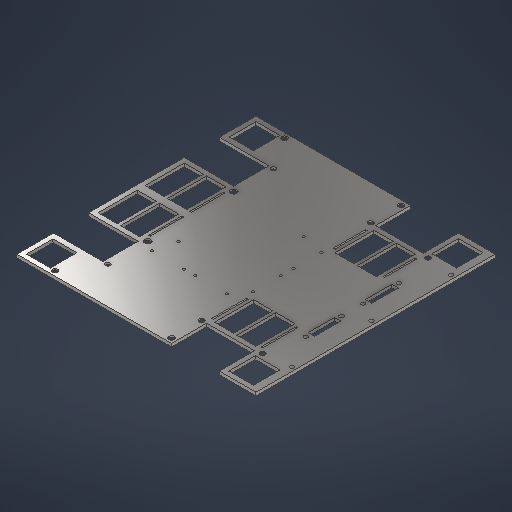
# Autodesk Inventor part: base
Saved by Autodesk Inventor 2026.2 (Build 302298010, 298A)
## iProperties
Created: 2026-04-27
Part Number: base
Material: Steel, Mild
Document SubType Name: Modeling
Designer: karol
Density: 7.85 g/cm^3
Appearance: Semi-Polished
Mass: 32.7977 g
Surface Area: 363.268 cm^2
Volume: 32.7977 cm^3
Author: karol
Autodesk Inventor part; units mm, degrees
ref_plane "YZ Plane" through (0, 0, 0) normal (1, 0, 0) x (0, 1, 0)
ref_plane "XZ Plane" through (0, 0, 0) normal (0, 1, 0) x (-1, 0, 0)
ref_plane "XY Plane" through (0, 0, 0) normal (0, 0, 1) x (1, 0, 0)
sketch "Szkic1" plane through (0, 0, 0) normal (0, 1, 0) x (-1, 0, 0)
  line L0 (0, 0) -> (150, 0)
  line L1 (150, 0) -> (150, -75)
  line L2 (150, -75) -> (0, -75)
  line L3 (0, -75) -> (0, 0)
  line L4 (53, -53) -> (23, -53)
  line L5 (23, -53) -> (23, -75)
  line L6 (23, -75) -> (53, -75)
  line L7 (53, -75) -> (53, -53)
  line L8 (23, -53) -> (20, -53)
  line L9 (20, -53) -> (20, -75)
  line L10 (20, -75) -> (23, -75)
  line L11 (23, -75) -> (23, -53)
  line L12 (20, -75) -> (0, -75)
  line L13 (0, -75) -> (0, -72)
  line L14 (0, -72) -> (20, -72)
  line L15 (20, -72) -> (20, -75)
  line L16 (20, -72) -> (5, -72)
  line L17 (5, -72) -> (5, -55.8)
  line L18 (5, -55.8) -> (20, -55.8)
  line L19 (20, -55.8) -> (20, -72)
  line L20 (150, 0) -> (147, 0)
  line L21 (147, 0) -> (147, -75)
  line L22 (147, -75) -> (150, -75)
  line L23 (150, -75) -> (150, 0)
  line L24 (147, -75) -> (53, -75)
  line L25 (53, -75) -> (53, -72)
  line L26 (53, -72) -> (147, -72)
  line L27 (147, -72) -> (147, -75)
  line L28 (53, -72) -> (56, -72)
  line L29 (56, -72) -> (56, -53)
  line L30 (56, -53) -> (53, -53)
  line L31 (53, -53) -> (53, -72)
  line L32 (147, -72) -> (132, -72)
  line L33 (132, -72) -> (132, -55.8)
  line L34 (132, -55.8) -> (147, -55.8)
  line L35 (147, -55.8) -> (147, -72)
  line L36 (56, -53) -> (20, -53)
  line L37 (20, -53) -> (20, -50)
  line L38 (20, -50) -> (56, -50)
  line L39 (56, -50) -> (56, -53)
  line L40 (51, -50) -> (39, -50)
  line L41 (39, -50) -> (39, -25.5)
  line L42 (39, -25.5) -> (51, -25.5)
  line L43 (51, -25.5) -> (51, -50)
  line L44 (25, -50) -> (37, -50)
  line L45 (37, -50) -> (37, -25.5)
  line L46 (37, -25.5) -> (25, -25.5)
  line L47 (25, -25.5) -> (25, -50)
  line L48 (147, 0) -> (115, 0)
  line L49 (115, 0) -> (115, -2.5)
  line L50 (115, -2.5) -> (147, -2.5)
  line L51 (147, -2.5) -> (147, 0)
  line L52 (147, -2.5) -> (135, -2.5)
  line L53 (135, -2.5) -> (135, -27)
  line L54 (135, -27) -> (147, -27)
  line L55 (147, -27) -> (147, -2.5)
  line L56 (133, -2.5) -> (121, -2.5)
  line L57 (121, -2.5) -> (121, -27)
  line L58 (121, -27) -> (133, -27)
  line L59 (133, -27) -> (133, -2.5)
  line L60 (150, -27) -> (116, -27)
  line L61 (116, -27) -> (116, -30)
  line L62 (116, -30) -> (150, -30)
  line L63 (150, -30) -> (150, -27)
  line L64 (150, -30) -> (149, -30)
  line L65 (149, -30) -> (149, -52)
  line L66 (149, -52) -> (150, -52)
  line L67 (150, -52) -> (150, -30)
  line L68 (149, -30) -> (119, -30)
  line L69 (119, -30) -> (119, -52)
  line L70 (119, -52) -> (149, -52)
  line L71 (149, -52) -> (149, -30)
  line L72 (116, -30) -> (119, -30)
  line L73 (119, -30) -> (119, -52)
  line L74 (119, -52) -> (116, -52)
  line L75 (116, -52) -> (116, -30)
  line L76 (116, -52) -> (150, -52)
  line L77 (150, -52) -> (150, -55)
  line L78 (150, -55) -> (116, -55)
  line L79 (116, -55) -> (116, -52)
  line L80 (150, 0) -> (150, 75)
  line L81 (150, 75) -> (0, 75)
  line L82 (0, 75) -> (0, 0)
  line L83 (53, 53) -> (23, 53)
  line L84 (23, 53) -> (23, 75)
  line L85 (23, 75) -> (53, 75)
  line L86 (53, 75) -> (53, 53)
  line L87 (23, 53) -> (20, 53)
  line L88 (20, 53) -> (20, 75)
  line L89 (20, 75) -> (23, 75)
  line L90 (23, 75) -> (23, 53)
  line L91 (20, 75) -> (0, 75)
  line L92 (0, 75) -> (0, 72)
  line L93 (0, 72) -> (20, 72)
  line L94 (20, 72) -> (20, 75)
  line L95 (20, 72) -> (5, 72)
  line L96 (5, 72) -> (5, 55.8)
  line L97 (5, 55.8) -> (20, 55.8)
  line L98 (20, 55.8) -> (20, 72)
  line L99 (147, 0) -> (147, 75)
  line L100 (147, 75) -> (150, 75)
  line L101 (150, 75) -> (150, 0)
  line L102 (147, 75) -> (53, 75)
  line L103 (53, 75) -> (53, 72)
  line L104 (53, 72) -> (147, 72)
  line L105 (147, 72) -> (147, 75)
  line L106 (53, 72) -> (56, 72)
  line L107 (56, 72) -> (56, 53)
  line L108 (56, 53) -> (53, 53)
  line L109 (53, 53) -> (53, 72)
  line L110 (147, 72) -> (132, 72)
  line L111 (132, 72) -> (132, 55.8)
  line L112 (132, 55.8) -> (147, 55.8)
  line L113 (147, 55.8) -> (147, 72)
  line L114 (56, 53) -> (20, 53)
  line L115 (20, 53) -> (20, 50)
  line L116 (20, 50) -> (56, 50)
  line L117 (56, 50) -> (56, 53)
  line L118 (51, 50) -> (39, 50)
  line L119 (39, 50) -> (39, 25.5)
  line L120 (39, 25.5) -> (51, 25.5)
  line L121 (51, 25.5) -> (51, 50)
  line L122 (25, 50) -> (37, 50)
  line L123 (37, 50) -> (37, 25.5)
  line L124 (37, 25.5) -> (25, 25.5)
  line L125 (25, 25.5) -> (25, 50)
  line L126 (115, 0) -> (115, 2.5)
  line L127 (115, 2.5) -> (147, 2.5)
  line L128 (147, 2.5) -> (147, 0)
  line L129 (147, 2.5) -> (135, 2.5)
  line L130 (135, 2.5) -> (135, 27)
  line L131 (135, 27) -> (147, 27)
  line L132 (147, 27) -> (147, 2.5)
  line L133 (133, 2.5) -> (121, 2.5)
  line L134 (121, 2.5) -> (121, 27)
  line L135 (121, 27) -> (133, 27)
  line L136 (133, 27) -> (133, 2.5)
  line L137 (150, 27) -> (116, 27)
  line L138 (116, 27) -> (116, 30)
  line L139 (116, 30) -> (150, 30)
  line L140 (150, 30) -> (150, 27)
  line L141 (150, 30) -> (149, 30)
  line L142 (149, 30) -> (149, 52)
  line L143 (149, 52) -> (150, 52)
  line L144 (150, 52) -> (150, 30)
  line L145 (149, 30) -> (119, 30)
  line L146 (119, 30) -> (119, 52)
  line L147 (119, 52) -> (149, 52)
  line L148 (149, 52) -> (149, 30)
  line L149 (116, 30) -> (119, 30)
  line L150 (119, 30) -> (119, 52)
  line L151 (119, 52) -> (116, 52)
  line L152 (116, 52) -> (116, 30)
  line L153 (116, 52) -> (150, 52)
  line L154 (150, 52) -> (150, 55)
  line L155 (150, 55) -> (116, 55)
  line L156 (116, 55) -> (116, 52)
  point P0 (5, -72)
  point P1 (20, -55.8)
  point P2 (147, -27)
  point P3 (147, -2.5)
  point P4 (5, 72)
  point P5 (147, 27)
  point P6 (147, 2.5)
  point P7 (121, -2.5)
  dimension "d0" = 150
  dimension "d1" = 75
  dimension "d2" = 30
  dimension "d3" = 22
  dimension "d4" = 23
  dimension "d5" = 3
  dimension "d6" = 3
  dimension "d7" = 15
  dimension "d8" = 16.2
  dimension "d9" = 3
  dimension "d10" = 3
  dimension "d11" = 3
  dimension "d12" = 15
  dimension "d13" = 16.2
  dimension "d14" = 3
  dimension "d15" = 12
  dimension "d16" = 24.5
  dimension "d17" = 12
  dimension "d18" = 24.5
  dimension "d19" = 2
  dimension "d20" = 2
  dimension "d21" = 32
  dimension "d22" = 2.5
  dimension "d23" = 12
  dimension "d24" = 24.5
  dimension "d25" = 12
  dimension "d26" = 24.5
  dimension "d27" = 2
  dimension "d28" = 36
  dimension "d29" = 34
  dimension "d30" = 3
  dimension "d31" = 1
  dimension "d32" = 22
  dimension "d33" = 30
  dimension "d34" = 22
  dimension "d35" = 3
  constraints: 314 end point, 61 symmetric about line, 40 parallel, 21 horizontal, 20 perpendicular, 18 point on line, 1 collinear
  measures "d0" distance of L1.end L2.end
  measures "d1" distance of L0.end L1.end
  measures "d2" distance of L6.end L5.end
  measures "d3" distance of L5.end L4.end
  measures "d4" distance between parallel lines of L3 L5
  measures "d5" distance of L10.end L9.end
  measures "d6" distance of L12.end L13.end
  measures "d7" distance of L17.end L18.end
  measures "d8" distance of L16.end L17.end
  measures "d9" distance of L22.end L21.end
  measures "d10" distance of L24.end L25.end
  measures "d11" distance of L30.end L29.end
  measures "d12" distance of L33.end L34.end
  measures "d13" distance of L32.end L33.end
  measures "d14" distance of L36.end L37.end
  measures "d15" distance of L41.end L42.end
  measures "d16" distance of L40.end L41.end
  measures "d17" distance of L46.end L45.end
  measures "d18" distance of L45.end L44.end
  measures "d19" distance between parallel lines of L31 L43
  measures "d20" distance between parallel lines of L47 L11
  measures "d21" distance of L50.end L49.end
  measures "d22" distance of L49.end L48.end
  measures "d23" distance of L54.end L53.end
  measures "d24" distance of L53.end L52.end
  measures "d25" distance of L58.end L57.end
  measures "d26" distance of L57.end L56.end
  measures "d27" distance between parallel lines of L53 L59
  measures "d28" distance of L37.end L38.end
  measures "d29" distance of L62.end L61.end
  measures "d30" distance of L61.end L60.end
  measures "d31" distance of L66.end L65.end
  measures "d32" distance of L65.end L64.end
  measures "d33" distance of L70.end L69.end
  measures "d34" distance of L69.end L68.end
  measures "d35" distance of L76.end L77.end
extrude "Wyciągnięcie proste1" add sketch "Szkic1" along normal blind 2 contours L82 L93 L96 L97 L88 L115 L116 L125 L124 L123 L119 L120 L121 L117 L107 L104 L111 L112 L99 L155 L156 L152 L138 L137 L134 L127 L126 L0 | L0 L49 L50 L57 L60 L61 L75 L79 L78 L21 L34 L33 L26 L29 L39 L38 L43 L42 L41 L45 L46 L47 L37 L9 L18 L17 L14 L3 | L126 L127 L99 L0 | L0 L21 L50 L49 | L14 L9 L2 L3 | L82 L81 L88 L93 | L99 L137 L80 L0 | L0 L1 L60 L21 | L9 L8 L5 L2 | L81 L84 L87 L88 | L1 L62 L21 L60 | L137 L99 L139 L80 | L21 L62 L61 L60 L58 L54 | L53 L60 L59 L50 | L131 L137 L135 L138 L139 L99 | L127 L136 L137 L130 | L7 L26 L21 L2 | L8 L37 L38 L39 L30 L4 | L81 L99 L104 L86 | L83 L108 L117 L116 L115 L87 | L1 L78 L21 L70 L66 | L143 L147 L99 L155 L80 | L21 L78 L79 L74 L70 | L69 L74 L75 L62 | L147 L151 L156 L155 L99 | L139 L152 L151 L146 | L21 L78 L1 L2 | L7 L30 L29 L26 | L81 L80 L155 L99 | L104 L107 L108 L86
sketch "Szkic2" plane through (0, 0, 0) normal (0, -1, 0) x (1, 0, 0)
  line L0 (-59, -69) -> (-53, -69)
  line L1 (-53, -69) -> (-53, -75)
  line L2 (-53, -75) -> (-59, -75)
  line L3 (-59, -75) -> (-59, -69)
  line L4 (-59, -69) -> (-53, -75) construction
  line L5 (-53, -69) -> (-59, -75) construction
  line L6 (-53, -53) -> (-53, -75) projected
  line L7 (-53, -75) -> (-150, -75) projected
  circle A0 centre (-56, -72) radius 1.75
  point P0 (0, 0)
  dimension "d38" = 6
  dimension "d39" = 6
  dimension "d40" = 3.5
  constraints: 12 end point, 2 collinear, 2 midpoint, 2 parallel, 1 centre point, 1 coincident, 1 horizontal, 1 perpendicular
  measures "d38" distance of L1.end L2.end
  measures "d39" distance of L0.end L1.end
  measures "d40" diameter of A0
extrude "Wyciągnięcie proste2" cut sketch "Szkic2" against normal blind 2 contours A0
sketch "Szkic3" plane through (0, 0, 0) normal (0, -1, 0) x (1, 0, 0)
  line L0 (-132, -75) -> (-126, -75)
  line L1 (-126, -75) -> (-126, -69)
  line L2 (-126, -69) -> (-132, -69)
  line L3 (-132, -69) -> (-132, -75)
  line L4 (-132, -75) -> (-126, -69) construction
  line L5 (-126, -75) -> (-132, -69) construction
  line L6 (-53, -75) -> (-150, -75) projected
  line L7 (-53, -53) -> (-53, -75) projected
  circle A0 centre (-129, -72) radius 1.75
  point P0 (0, 0)
  point P1 (-126, -72)
  dimension "d43" = 6
  dimension "d44" = 6
  dimension "d45" = 73
  dimension "d46" = 3.5
  constraints: 12 end point, 3 midpoint, 2 parallel, 1 centre point, 1 coincident, 1 collinear, 1 horizontal, 1 perpendicular
  measures "d43" distance of L2.end L1.end
  measures "d44" distance of L1.end L0.end
  measures "d45" distance from line of point (-126, -72) L7
  measures "d46" diameter of A0
extrude "Wyciągnięcie proste3" cut sketch "Szkic3" against normal blind 2 contours A0
sketch "Szkic4" plane through (0, 0, 0) normal (0, -1, 0) x (1, 0, 0)
  line L0 (-59, 69) -> (-53, 69)
  line L1 (-53, 69) -> (-53, 75)
  line L2 (-53, 75) -> (-59, 75)
  line L3 (-59, 75) -> (-59, 69)
  line L4 (-59, 69) -> (-53, 75) construction
  line L5 (-53, 69) -> (-59, 75) construction
  line L6 (-150, 75) -> (-53, 75) projected
  line L7 (-53, 75) -> (-53, 53) projected
  circle A0 centre (-56, 72) radius 1.75
  point P0 (0, 0)
  dimension "d49" = 6
  dimension "d50" = 6
  dimension "d51" = 3.5
  constraints: 12 end point, 2 collinear, 2 midpoint, 2 parallel, 1 centre point, 1 coincident, 1 horizontal, 1 perpendicular
  measures "d49" distance of L2.end L1.end
  measures "d50" distance of L1.end L0.end
  measures "d51" diameter of A0
extrude "Wyciągnięcie proste4" cut sketch "Szkic4" against normal blind 2 contours A0
sketch "Szkic5" plane through (0, 0, 0) normal (0, -1, 0) x (1, 0, 0)
  line L0 (-132, 75) -> (-126, 75)
  line L1 (-126, 75) -> (-126, 69)
  line L2 (-126, 69) -> (-132, 69)
  line L3 (-132, 69) -> (-132, 75)
  line L4 (-132, 75) -> (-126, 69) construction
  line L5 (-126, 75) -> (-132, 69) construction
  line L6 (-150, 75) -> (-53, 75) projected
  line L7 (-53, 75) -> (-53, 53) projected
  circle A0 centre (-129, 72) radius 1.75
  point P0 (0, 0)
  dimension "d54" = 6
  dimension "d55" = 6
  dimension "d56" = 73
  dimension "d57" = 3.5
  constraints: 12 end point, 2 midpoint, 2 parallel, 1 centre point, 1 coincident, 1 collinear, 1 horizontal, 1 perpendicular
  measures "d54" distance of L1.end L2.end
  measures "d55" distance of L0.end L1.end
  measures "d56" distance between parallel lines of L7 L1
  measures "d57" diameter of A0
extrude "Wyciągnięcie proste5" cut sketch "Szkic5" against normal blind 2 contours A0
sketch "Szkic6" plane through (0, 0, 0) normal (0, -1, 0) x (1, 0, 0)
  circle A0 centre (-116, -52) radius 1.5
  line L0 (-119, -52) -> (-119, -30) projected
  line L1 (-150, -52) -> (-119, -52) projected
  point P0 (0, 0)
  dimension "d60" = 3
  dimension "d61" = 3
  dimension "d62" = 0
  constraints: 1 centre point
  measures "d60" diameter of A0
  measures "d61" distance from line of A0.centre L0
  measures "d62" distance from line of L1 A0.centre
extrude "Wyciągnięcie proste6" cut sketch "Szkic6" against normal blind 2
sketch "Szkic7" plane through (0, 0, 0) normal (0, -1, 0) x (1, 0, 0)
  circle A0 centre (-116, 52) radius 1.5
  line L0 (-119, 52) -> (-150, 52) projected
  line L1 (-119, 30) -> (-119, 52) projected
  point P0 (0, 0)
  dimension "d65" = 3
  dimension "d66" = 0
  dimension "d67" = 3
  constraints: 1 centre point
  measures "d65" diameter of A0
  measures "d66" distance from line of A0.centre L0
  measures "d67" distance from line of L1 A0.centre
extrude "Wyciągnięcie proste7" cut sketch "Szkic7" against normal blind 2
sketch "Szkic8" plane through (0, 2, 0) normal (0, 1, 0) x (1, 0, 0)
  line L0 (-119, 52) -> (-119, 30) projected
  line L1 (-119, 30) -> (-113, 30)
  line L2 (-113, 30) -> (-113, 24)
  line L3 (-113, 24) -> (-119, 24)
  line L4 (-119, 24) -> (-119, 30)
  circle A0 centre (-116, 27) radius 2
  point P0 (0, 0)
  dimension "d70" = 6
  dimension "d71" = 6
  dimension "d72" = 4
  constraints: 8 end point, 2 parallel, 1 centre point, 1 horizontal, 1 perpendicular
  measures "d70" distance of L2.end L3.end
  measures "d71" distance of L1.end L2.end
  measures "d72" diameter of A0
extrude "Wyciągnięcie proste8" cut sketch "Szkic8" against normal blind 2 contours A0
sketch "Szkic9" plane through (0, 0, 0) normal (0, -1, 0) x (1, 0, 0)
  circle A0 centre (-116, 27) radius 2
  line L0 (-150, 30) -> (-119, 30) projected
  line L1 (-119, 30) -> (-119, 52) projected
  point P0 (0, 0)
  dimension "d75" = 4
  dimension "d76" = 3
  dimension "d77" = 3
  constraints: 1 centre point
  measures "d75" diameter of A0
  measures "d76" distance from line of A0.centre L0
  measures "d77" distance from line of A0.centre L1
extrude "Wyciągnięcie proste9" cut sketch "Szkic9" against normal blind 2
sketch "Szkic10" plane through (0, 0, 0) normal (0, -1, 0) x (1, 0, 0)
  line L0 (-53, 75) -> (-53, 53) projected
  line L1 (-53, 53) -> (-56, 53)
  line L2 (-56, 53) -> (-56, 56)
  line L3 (-56, 56) -> (-53, 56)
  line L4 (-53, 56) -> (-53, 53)
  line L5 (-53, 56) -> (-59, 56)
  line L6 (-59, 56) -> (-59, 50)
  line L7 (-59, 50) -> (-53, 50)
  line L8 (-53, 50) -> (-53, 56)
  circle A0 centre (-56, 53) radius 2
  point P0 (0, 0)
  dimension "d80" = 3
  dimension "d81" = 3
  dimension "d82" = 6
  dimension "d83" = 6
  dimension "d84" = 4
  constraints: 16 end point, 4 parallel, 2 horizontal, 2 perpendicular, 1 centre point, 1 coincident
  measures "d80" distance of L2.end L3.end
  measures "d81" distance of L1.end L2.end
  measures "d82" distance of L7.end L6.end
  measures "d83" distance of L6.end L5.end
  measures "d84" diameter of A0
hole "Otwór1" at (-56, 0, 53) direction (0, 1, 0) diameter 3.3 depth 2 tip angle 118 countersink diameter 6 countersink angle 90
sketch "Szkic11" plane through (0, 0, 0) normal (0, -1, 0) x (1, 0, 0)
  circle A0 centre (-116, 27) radius 2 projected
  circle A1 centre (-116, 27) radius 0.6329
  circle A2 centre (-116, 52) radius 1.5 projected
  circle A3 centre (-116, 52) radius 0.49
  circle A4 centre (-129, 72) radius 1.75 projected
  circle A5 centre (-129, 72) radius 0.3159
  circle A6 centre (-56, 72) radius 1.75 projected
  circle A7 centre (-56, 72) radius 1.0716
  circle A8 centre (-116, -27) radius 2 projected
  circle A9 centre (-116, -27) radius 0.6329
  circle A10 centre (-129, -72) radius 1.75 projected
  circle A11 centre (-129, -72) radius 0.3159
  circle A12 centre (-116, -52) radius 1.5 projected
  circle A13 centre (-116, -52) radius 0.49
  circle A14 centre (-56, -72) radius 1.75 projected
  circle A15 centre (-56, -72) radius 1.0716
  point P0 (0, 0)
  constraints: 8 centre point, 8 coincident
hole "Otwór2" at (-129, 0, 72) at (-56, 0, 72) at (-56, 0, -72) at (-129, 0, -72) direction (0, 1, 0) diameter 3.3 depth 2 tip angle 118 countersink diameter 6 countersink angle 90
hole "Otwór3" at (-116, 0, 52) at (-116, 0, -52) at (-56, 0, 72) at (-56, 0, -72) direction (0, 1, 0) diameter 2.3 depth 2 tip angle 118 countersink diameter 4.5 countersink angle 90
hole "Otwór4" at (-116, 0, 27) at (-116, 0, -27) direction (0, 1, 0) diameter 3.3 depth 2 tip angle 118 countersink diameter 6.3 countersink angle 90
sketch "Szkic12" plane through (0, 0, 0) normal (0, -1, 0) x (1, 0, 0)
  line L0 (-53, -53) -> (-53, -75) projected
  line L1 (-53, -53) -> (-56, -53)
  line L2 (-56, -53) -> (-56, -56)
  line L3 (-56, -56) -> (-53, -56)
  line L4 (-53, -56) -> (-53, -53)
  line L5 (-53, -56) -> (-59, -56)
  line L6 (-59, -56) -> (-59, -50)
  line L7 (-59, -50) -> (-53, -50)
  line L8 (-53, -50) -> (-53, -56)
  circle A0 centre (-56, -53) radius 0.9499
  point P0 (0, 0)
  dimension "d113" = 3
  dimension "d114" = 3
  dimension "d115" = 6
  dimension "d116" = 6
  constraints: 16 end point, 4 parallel, 2 horizontal, 2 perpendicular, 1 centre point, 1 coincident
  measures "d113" distance of L3.end L2.end
  measures "d114" distance of L2.end L1.end
  measures "d115" distance of L6.end L7.end
  measures "d116" distance of L5.end L6.end
hole "Otwór5" at (-56, 0, -53) direction (0, 1, 0) diameter 3.3 depth 2 tip angle 118 countersink diameter 6 countersink angle 90
sketch "Szkic13" plane through (0, 0, 0) normal (0, -1, 0) x (1, 0, 0)
  line L0 (-23, 53) -> (-23, 75) projected
  line L1 (-23, 53) -> (-15, 53)
  line L2 (-15, 53) -> (-15, 50)
  line L3 (-15, 50) -> (-23, 50)
  line L4 (-23, 50) -> (-23, 53)
  line L5 (-23, 50) -> (-15, 50)
  line L6 (-15, 50) -> (-15, 54.8)
  line L7 (-15, 54.8) -> (-23, 54.8)
  line L8 (-23, 54.8) -> (-23, 50)
  line L9 (-23, 50) -> (-15, 50)
  line L10 (-15, 50) -> (-15, 48.8)
  line L11 (-15, 48.8) -> (-23, 48.8)
  line L12 (-23, 48.8) -> (-23, 50)
  circle A0 centre (-19, 51.8) radius 0.8808
  point P0 (0, 0)
  dimension "d124" = 8
  dimension "d125" = 3
  dimension "d126" = 4.8
  dimension "d127" = 1.2
  dimension "d128" = 3
  dimension "d129" = 4
  constraints: 24 end point, 6 parallel, 3 horizontal, 3 perpendicular, 1 centre point
  measures "d124" distance of L2.end L3.end
  measures "d125" distance of L1.end L2.end
  measures "d126" distance of L6.end L5.end
  measures "d127" distance of L9.end L10.end
  measures "d128" distance from line of L11 A0.centre
  measures "d129" distance from line of L2 A0.centre
hole "Otwór6" at (-19, 0, 51.8) direction (0, 1, 0) diameter 3.3 depth 2 tip angle 118 countersink diameter 6.3 countersink angle 90
sketch "Szkic14" plane through (0, 0, 0) normal (0, -1, 0) x (1, 0, 0)
  circle A0 centre (-19, 51.8) radius 1.65 projected
  circle A1 centre (-19, 51.8) radius 3.15 projected
  circle A2 centre (-19, 51.8) radius 3.15 projected
  line L0 (-133, -2.5) -> (-133, -27) projected
  line L1 (-121, -2.5) -> (-133, -2.5) projected
  line L2 (-121, -27) -> (-121, -2.5) projected
  line L3 (-133, -27) -> (-121, -27) projected
  line L4 (-135, 2.5) -> (-135, 27) projected
  line L5 (-147, 2.5) -> (-135, 2.5) projected
  line L6 (-147, 27) -> (-147, 2.5) projected
  line L7 (-135, 27) -> (-147, 27) projected
  line L8 (-37, -50) -> (-25, -50) projected
  line L9 (-37, -25.5) -> (-37, -50) projected
  line L10 (-25, -25.5) -> (-37, -25.5) projected
  line L11 (-25, -50) -> (-25, -25.5) projected
  line L12 (-39, -50) -> (-39, -25.5) projected
  line L13 (-51, -50) -> (-39, -50) projected
  line L14 (-51, -25.5) -> (-51, -50) projected
  line L15 (-39, -25.5) -> (-51, -25.5) projected
  line L16 (-51, 50) -> (-51, 25.5) projected
  line L17 (-39, 50) -> (-51, 50) projected
  line L18 (-39, 25.5) -> (-39, 50) projected
  line L19 (-51, 25.5) -> (-39, 25.5) projected
  line L20 (-37, 50) -> (-37, 25.5) projected
  line L21 (-25, 50) -> (-37, 50) projected
  line L22 (-25, 25.5) -> (-25, 50) projected
  line L23 (-37, 25.5) -> (-25, 25.5) projected
  line L24 (-133, 2.5) -> (-121, 2.5) projected
  line L25 (-133, 27) -> (-133, 2.5) projected
  line L26 (-121, 27) -> (-133, 27) projected
  line L27 (-121, 2.5) -> (-121, 27) projected
  line L28 (-20, 72) -> (-20, 55.8) projected
  line L29 (-5, 72) -> (-20, 72) projected
  line L30 (-5, 55.8) -> (-5, 72) projected
  line L31 (-20, 55.8) -> (-5, 55.8) projected
  line L32 (-132, -72) -> (-132, -55.8) projected
  arc A3 (-129, -75) -> (-132, -72) centre (-129, -72) ccw projected
  line L33 (-56, -75) -> (-129, -75) projected
  arc A4 (-53, -72) -> (-56, -75) centre (-56, -72) ccw projected
  line L34 (-53, -53) -> (-53, -72) projected
  circle A5 centre (-56, -53) radius 3 projected
  line L35 (-23, -53) -> (-53, -53) projected
  line L36 (-23, -75) -> (-23, -53) projected
  line L37 (0, -75) -> (-23, -75) projected
  line L38 (0, 75) -> (0, -75) projected
  line L39 (-23, 75) -> (0, 75) projected
  line L40 (-23, 53) -> (-23, 75) projected
  line L41 (-53, 53) -> (-23, 53) projected
  circle A6 centre (-56, 53) radius 3 projected
  line L42 (-53, 72) -> (-53, 53) projected
  arc A7 (-56, 75) -> (-53, 72) centre (-56, 72) ccw projected
  line L43 (-129, 75) -> (-56, 75) projected
  arc A8 (-132, 72) -> (-129, 75) centre (-129, 72) ccw projected
  line L44 (-132, 55.8) -> (-132, 72) projected
  line L45 (-147, 55.8) -> (-132, 55.8) projected
  line L46 (-147, 72) -> (-147, 55.8) projected
  line L47 (-132, 72) -> (-147, 72) projected
  arc A9 (-129, 75) -> (-132, 72) centre (-129, 72) ccw projected
  line L48 (-150, 75) -> (-129, 75) projected
  line L49 (-150, 52) -> (-150, 75) projected
  line L50 (-119, 52) -> (-150, 52) projected
  line L51 (-119, 30) -> (-119, 52) projected
  line L52 (-150, 30) -> (-119, 30) projected
  line L53 (-150, -30) -> (-150, 30) projected
  line L54 (-119, -30) -> (-150, -30) projected
  line L55 (-119, -52) -> (-119, -30) projected
  line L56 (-150, -52) -> (-119, -52) projected
  line L57 (-150, -75) -> (-150, -52) projected
  line L58 (-129, -75) -> (-150, -75) projected
  arc A10 (-132, -72) -> (-129, -75) centre (-129, -72) ccw projected
  line L59 (-147, -72) -> (-132, -72) projected
  line L60 (-147, -55.8) -> (-147, -72) projected
  line L61 (-132, -55.8) -> (-147, -55.8) projected
  line L62 (-147, -27) -> (-135, -27) projected
  line L63 (-147, -2.5) -> (-147, -27) projected
  line L64 (-135, -2.5) -> (-147, -2.5) projected
  line L65 (-135, -27) -> (-135, -2.5) projected
  line L66 (-20, -72) -> (-5, -72) projected
  line L67 (-20, -55.8) -> (-20, -72) projected
  line L68 (-5, -55.8) -> (-20, -55.8) projected
  line L69 (-5, -72) -> (-5, -55.8) projected
  circle A11 centre (-116, 52) radius 2.25 projected
  circle A12 centre (-116, -52) radius 2.25 projected
  circle A13 centre (-116, 27) radius 3.15 projected
  circle A14 centre (-116, -27) radius 3.15 projected
  line L70 (0, 0) -> (-43.2972, 0)
  circle A15 centre (-19, -51.8) radius 3.15
  constraints: 2 end point, 2 horizontal alignment, 2 symmetric about line, 1 centre point, 1 horizontal, 1 other
hole "Otwór7" at (-19, 0, -51.8) direction (0, 1, 0) diameter 3.3 depth 2 tip angle 118 countersink diameter 6.3 countersink angle 90
sketch "Sketch27" plane through (0, 2, 0) normal (0, 1, 0) x (1, 0, 0)
  circle A0 centre (-2.5, -50) radius 1.25
  circle A1 centre (-2.5, 0) radius 1.25
  circle A2 centre (-2.5, 50) radius 1.25
  line L0 (-23, -75) -> (0, -75) projected
  line L1 (0, 75) -> (-23, 75) projected
  line L2 (0, -75) -> (0, 75) projected
  point P0 (0, 0)
  dimension "d253" = 2.5
  dimension "d254" = 2.5
  dimension "d256" = 2.5
  dimension "d257" = 25
  dimension "d258" = 25
  dimension "d259" = 2.5
  dimension "d260" = 2.5
  dimension "d262" = 2.5
  dimension "d265" = 75
  constraints: 3 centre point
  measures "d253" diameter of A0
  measures "d254" diameter of A1
  measures "d256" diameter of A2
  measures "d257" distance from line of L0 A0.centre
  measures "d258" distance from line of L1 A2.centre
  measures "d259" distance from line of L2 A2.centre
  measures "d260" distance from line of L2 A0.centre
  measures "d262" distance from line of L2 A1.centre
  measures "d265" distance from line of L0 A1.centre
extrude "Extrusion26" cut sketch "Sketch27" against normal blind 2
thread "Thread7" size "M3x0.5" class "6H" standard "ANSI Metric M Profile" full length
thread "Thread8" size "M3x0.5" class "6H" standard "ANSI Metric M Profile" full length
thread "Thread9" size "M3x0.5" class "6H" standard "ANSI Metric M Profile" full length
sketch "Sketch29" plane through (0, 2, 0) normal (0, 1, 0) x (1, 0, 0)
  circle A0 centre (-109.5, -30.75) radius 0.8
  circle A1 centre (-89.5, -30.75) radius 0.8
  line L0 (-119, -30) -> (-119, -52) projected
  line L1 (-150, -75) -> (-53, -75) projected
  point P0 (0, 0)
  point P1 (-119, -41)
  dimension "d280" = 1.6
  dimension "d281" = 1.6
  dimension "d282" = 9.5
  dimension "d283" = 29.5
  dimension "d284" = 44.25
  dimension "d285" = 44.25
  constraints: 2 centre point, 1 midpoint
  measures "d280" diameter of A0
  measures "d281" diameter of A1
  measures "d282" distance from line of L0 A0.centre
  measures "d283" horizontal distance of point (-119, -41) A1.centre
  measures "d284" distance from line of L1 A0.centre
  measures "d285" distance from line of L1 A1.centre
extrude "Extrusion27" cut sketch "Sketch29" against normal blind 2
thread "Thread10" size "M2x0.4" class "6H" standard "ANSI Metric M Profile" full length
thread "Thread11" size "M2x0.4" class "6H" standard "ANSI Metric M Profile" full length
sketch "Sketch30" plane through (0, 2, 0) normal (0, 1, 0) x (1, 0, 0)
  circle A0 centre (-82.5, -30.75) radius 0.8
  circle A1 centre (-62.5, -30.75) radius 0.8
  line L0 (-119, -30) -> (-119, -52) projected
  line L1 (-150, -75) -> (-53, -75) projected
  point P0 (0, 0)
  dimension "d292" = 1.6
  dimension "d293" = 1.6
  dimension "d294" = 36.5
  dimension "d295" = 56.5
  dimension "d296" = 44.25
  dimension "d297" = 44.25
  constraints: 2 centre point
  measures "d292" diameter of A0
  measures "d293" diameter of A1
  measures "d294" distance from line of L0 A0.centre
  measures "d295" distance from line of L0 A1.centre
  measures "d296" distance from line of L1 A1.centre
  measures "d297" distance from line of L1 A0.centre
extrude "Extrusion28" cut sketch "Sketch30" against normal blind 2
thread "Thread12" size "M2x0.4" class "6H" standard "ANSI Metric M Profile" full length
thread "Thread13" size "M2x0.4" class "6H" standard "ANSI Metric M Profile" full length
sketch "Szkic31" plane through (0, 2, 0) normal (0, 1, 0) x (1, 0, 0)
  circle A0 centre (-55.5, -21.5) radius 0.8
  circle A1 centre (-55.5, -4) radius 0.8
  circle A2 centre (-55.5, 4) radius 0.8
  circle A3 centre (-55.5, 21.5) radius 0.8
  line L0 (-53, -53) -> (-23, -53) projected
  line L1 (-53, -75) -> (-53, -53) projected
  line L2 (-23, -53) -> (-23, -75) projected
  line L3 (-23, 53) -> (-53, 53) projected
  point P0 (0, 0)
  dimension "d304" = 1.6
  dimension "d305" = 1.6
  dimension "d306" = 1.6
  dimension "d307" = 1.6
  dimension "d308" = 31.5
  dimension "d310" = 32.5
  dimension "d311" = 32.5
  dimension "d312" = 32.5
  dimension "d313" = 32.5
  dimension "d314" = 31.5
  dimension "d315" = 49
  dimension "d316" = 49
  constraints: 4 centre point
  measures "d304" diameter of A0
  measures "d305" diameter of A1
  measures "d306" diameter of A2
  measures "d307" diameter of A3
  measures "d308" distance from line of L0 A0.centre
  measures "d310" distance from line of A0.centre L2
  measures "d311" distance from line of L2 A1.centre
  measures "d312" distance from line of L2 A2.centre
  measures "d313" distance from line of L2 A3.centre
  measures "d314" distance from line of L3 A3.centre
  measures "d315" distance from line of A1.centre L0
  measures "d316" distance from line of A2.centre L3
extrude "Wyciągnięcie proste29" cut sketch "Szkic31" against normal blind 2
thread "Gwint14" size "M2x0.4" class "6H" standard "ANSI Metric M Profile" full length
thread "Gwint15" size "M2x0.4" class "6H" standard "ANSI Metric M Profile" full length
thread "Gwint16" size "M2x0.4" class "6H" standard "ANSI Metric M Profile" full length
thread "Thread17" size "M2x0.4" class "6H" standard "ANSI Metric M Profile" full length
sketch "Szkic32" plane through (0, 2, 0) normal (0, 1, 0) x (1, 0, 0)
  circle A0 centre (-14, -25) radius 1.25
  circle A1 centre (-14, 25) radius 1.25
  line L0 (-23, -75) -> (0, -75) projected
  line L1 (0, -75) -> (0, 75) projected
  line L2 (0, 75) -> (-23, 75) projected
  circle A2 centre (-14, -11) radius 1.25
  circle A3 centre (-14, 11) radius 1.25
  point P0 (0, 0)
  point P1 (0, -13.5262)
  point P2 (0, -15.0262)
  dimension "d327" = 2.5
  dimension "d328" = 2.5
  dimension "d329" = 50
  dimension "d330" = 14
  dimension "d331" = 14
  dimension "d332" = 50
  dimension "d333" = 2.5
  dimension "d334" = 2.5
  dimension "d335" = 14
  dimension "d336" = 14
  dimension "d337" = 14
  dimension "d338" = 14
  constraints: 4 centre point
  measures "d327" diameter of A0
  measures "d328" diameter of A1
  measures "d329" distance from line of L0 A0.centre
  measures "d330" distance from line of L1 A0.centre
  measures "d331" distance from line of L1 A1.centre
  measures "d332" distance from line of L2 A1.centre
  measures "d333" diameter of A2
  measures "d334" diameter of A3
  measures "d335" distance from line of L1 A2.centre
  measures "d336" distance from line of L1 A3.centre
  measures "d337" distance of A1.centre A3.centre
  measures "d338" distance of A0.centre A2.centre
extrude "Wyciągnięcie proste30" cut sketch "Szkic32" against normal blind 2
sketch "Szkic33" plane through (0, 2, 0) normal (0, 1, 0) x (1, 0, 0)
  line L0 (-5, 55.8) -> (-20, 55.8) projected
  line L1 (-20, 55.8) -> (-5, 55.8)
  line L2 (-5, 55.8) -> (-5, 55.4)
  line L3 (-5, 55.4) -> (-20, 55.4)
  line L4 (-20, 55.4) -> (-20, 55.8)
  line L5 (-5, 55.4) -> (-4.6, 55.4)
  line L6 (-4.6, 55.4) -> (-4.6, 72)
  line L7 (-4.6, 72) -> (-5, 72)
  line L8 (-5, 72) -> (-5, 55.4)
  line L9 (-20, -72) -> (-20, -55.8) projected
  line L10 (-20, -55.8) -> (-5, -55.8)
  line L11 (-5, -55.8) -> (-5, -55.4)
  line L12 (-5, -55.4) -> (-20, -55.4)
  line L13 (-20, -55.4) -> (-20, -55.8)
  line L14 (-5, -55.4) -> (-4.6, -55.4)
  line L15 (-4.6, -55.4) -> (-4.6, -72)
  line L16 (-4.6, -72) -> (-5, -72)
  line L17 (-5, -72) -> (-5, -55.4)
  line L18 (-147, -72) -> (-147, -55.8) projected
  line L19 (-147, -55.8) -> (-132, -55.8)
  line L20 (-132, -55.8) -> (-132, -55.4)
  line L21 (-132, -55.4) -> (-147, -55.4)
  line L22 (-147, -55.4) -> (-147, -55.8)
  line L23 (-132, -72) -> (-132, -55.4)
  line L24 (-132, 55.8) -> (-147, 55.8) projected
  line L25 (-147, 55.8) -> (-132, 55.8)
  line L26 (-132, 55.8) -> (-132, 55.4)
  line L27 (-132, 55.4) -> (-147, 55.4)
  line L28 (-147, 55.4) -> (-147, 55.8)
  point P0 (0, 0)
  dimension "d341" = 0.4
  dimension "d342" = 0.4
  dimension "d343" = 0.4
  dimension "d344" = 0.4
  dimension "d345" = 0.4
  constraints: 50 end point, 12 parallel, 6 horizontal, 6 perpendicular
  measures "d341" distance of L1.end L2.end
  measures "d342" distance of L7.end L6.end
  measures "d343" distance of L11.end L10.end
  measures "d344" distance of L15.end L16.end
  measures "d345" distance of L20.end L19.end
extrude "Wyciągnięcie proste31" cut sketch "Szkic33" against normal blind 2
sketch "Szkic34" plane through (0, 2, 0) normal (0, 1, 0) x (1, 0, 0)
  circle A0 centre (-14, 25) radius 1.25 projected
  circle A1 centre (-14, 11) radius 1.25 projected
  line L0 (-14, 25) -> (-14, 11)
  line L1 (-14, 11) -> (-14, 18)
  line L2 (-16, 9.75) -> (-16, 26.25)
  line L3 (-16, 26.25) -> (-12, 26.25)
  line L4 (-12, 26.25) -> (-12, 9.75)
  line L5 (-12, 9.75) -> (-16, 9.75)
  line L6 (-16, 9.75) -> (-12, 26.25) construction
  line L7 (-16, 26.25) -> (-12, 9.75) construction
  circle A2 centre (-14, -11) radius 1.25 projected
  circle A3 centre (-14, -25) radius 1.25 projected
  line L8 (-14, -11) -> (-14, -25)
  line L9 (-14, -25) -> (-14, -18)
  line L10 (-16, -26.25) -> (-16, -9.75)
  line L11 (-16, -9.75) -> (-12, -9.75)
  line L12 (-12, -9.75) -> (-12, -26.25)
  line L13 (-12, -26.25) -> (-16, -26.25)
  line L14 (-16, -26.25) -> (-12, -9.75) construction
  line L15 (-16, -9.75) -> (-12, -26.25) construction
  point P0 (0, 0)
  dimension "d387" = 4
  dimension "d388" = 4
  dimension "d389" = 4
  dimension "d390" = 4
  constraints: 32 end point, 6 midpoint, 4 parallel, 2 perpendicular, 2 vertical
  measures "d387" distance of L10.end L11.end
  measures "d388" distance of L12.end L10.start
  measures "d389" distance of L4.end L2.start
  measures "d390" distance of L2.end L3.end
extrude "Wyciągnięcie proste32" cut sketch "Szkic34" against normal blind 2
sketch "Szkic35" plane through (0, 2, 0) normal (0, 1, 0) x (1, 0, 0)
  circle A0 centre (-14.5, 29.25) radius 1.25
  circle A1 centre (-14.5, 6.75) radius 1.25
  line L0 (-16, 9.75) -> (-16, 26.25) projected
  line L1 (-12, 9.75) -> (-16, 9.75) projected
  line L2 (-16, 26.25) -> (-12, 26.25) projected
  point P0 (0, 0)
  point P1 (-14, 9.75)
  point P2 (-14, 26.25)
  dimension "d351" = 2.5
  dimension "d352" = 2.5
  dimension "d353" = 1.5
  dimension "d354" = 1.5
  dimension "d355" = 3
  dimension "d356" = 3
  constraints: 2 centre point, 2 midpoint
  measures "d351" diameter of A0
  measures "d352" diameter of A1
  measures "d353" distance from line of L0 A1.centre
  measures "d354" distance from line of A0.centre L0
  measures "d355" vertical distance of point (-14, 9.75) A1.centre
  measures "d356" vertical distance of point (-14, 26.25) A0.centre
extrude "Wyciągnięcie proste33" cut sketch "Szkic35" against normal blind 2
thread "Gwint18" size "M3x0.5" class "6H" standard "ANSI Metric M Profile" full length
thread "Gwint19" size "M3x0.5" class "6H" standard "ANSI Metric M Profile" full length
sketch "Szkic36" plane through (0, 2, 0) normal (0, 1, 0) x (1, 0, 0)
  circle A0 centre (-14.5, -6.75) radius 1.3
  circle A1 centre (-14.5, -29.25) radius 1.25
  line L0 (-12, -26.25) -> (-16, -26.25) projected
  line L1 (-16, -26.25) -> (-16, -9.75) projected
  line L2 (-16, -9.75) -> (-12, -9.75) projected
  point P0 (0, 0)
  point P1 (-14, -26.25)
  point P2 (-14, -9.75)
  dimension "d363" = 2.6
  dimension "d364" = 2.5
  dimension "d365" = 3
  dimension "d366" = 1.5
  dimension "d367" = 1.5
  dimension "d368" = 3
  constraints: 2 centre point, 2 midpoint
  measures "d363" diameter of A0
  measures "d364" diameter of A1
  measures "d365" vertical distance of point (-14, -26.25) A1.centre
  measures "d366" distance from line of L1 A1.centre
  measures "d367" distance from line of L1 A0.centre
  measures "d368" vertical distance of point (-14, -9.75) A0.centre
extrude "Wyciągnięcie proste34" cut sketch "Szkic36" against normal blind 2
thread "Gwint20" size "M3x0.5" class "6H" standard "ANSI Metric M Profile" full length
thread "Gwint21" size "M3x0.5" class "6H" standard "ANSI Metric M Profile" full length
sketch "Sketch37" plane through (0, 2, 0) normal (0, 1, 0) x (1, 0, 0)
  circle A0 centre (-106.125, -17.575) radius 0.8
  line L0 (-150, -30) -> (-119, -30) projected
  line L1 (-119, -30) -> (-119, -52) projected
  circle A1 centre (-69.523, 24.496) radius 0.8
  point P0 (0, 0)
  dimension "d375" = 1.6
  dimension "d376" = 12.425
  dimension "d377" = 12.875
  dimension "d378" = 1.6
  dimension "d379" = 36.602
  dimension "d380" = 42.071
  constraints: 2 centre point
  measures "d375" diameter of A0
  measures "d376" distance from line of A0.centre L0
  measures "d377" distance from line of L1 A0.centre
  measures "d378" diameter of A1
  measures "d379" horizontal distance of A0.centre A1.centre
  measures "d380" vertical distance of A1.centre A0.centre
extrude "Extrusion35" cut sketch "Sketch37" against normal blind 2
thread "Thread22" size "M2x0.4" class "6H" standard "ANSI Metric M Profile" full length
thread "Thread23" size "M2x0.4" class "6H" standard "ANSI Metric M Profile" full length
sketch "Szkic38" plane through (0, 2, 0) normal (0, 1, 0) x (1, 0, 0)
  line L0 (-53, -26.75) -> (-54, -26.75)
  line L1 (-54, -26.75) -> (-54, -48.75)
  line L2 (-54, -48.75) -> (-53, -48.75)
  line L3 (-53, -48.75) -> (-53, -26.75)
  line L4 (-51, -25.5) -> (-39, -25.5) projected
  line L5 (-39, -50) -> (-51, -50) projected
  line L6 (-23, -26.75) -> (-22, -26.75)
  line L7 (-22, -26.75) -> (-22, -48.75)
  line L8 (-22, -48.75) -> (-23, -48.75)
  line L9 (-23, -48.75) -> (-23, -26.75)
  line L10 (-37, -25.5) -> (-25, -25.5) projected
  line L11 (-51, -50) -> (-51, -25.5) projected
  line L12 (-25, -25.5) -> (-25, -50) projected
  line L13 (-53, 47.75) -> (-54, 47.75)
  line L14 (-54, 47.75) -> (-54, 27.75)
  line L15 (-54, 27.75) -> (-53, 27.75)
  line L16 (-53, 27.75) -> (-53, 47.75)
  line L17 (-23, 47.75) -> (-22, 47.75)
  line L18 (-22, 47.75) -> (-22, 27.75)
  line L19 (-22, 27.75) -> (-23, 27.75)
  line L20 (-23, 27.75) -> (-23, 47.75)
  line L21 (-51, 50) -> (-39, 50) projected
  line L22 (-37, 50) -> (-25, 50) projected
  line L23 (-25, 50) -> (-25, 25.5) projected
  line L24 (-51, 25.5) -> (-51, 50) projected
  line L25 (-119, 2.5) -> (-118, 2.5)
  line L26 (-118, 2.5) -> (-118, 23.5)
  line L27 (-118, 23.5) -> (-119, 23.5)
  line L28 (-119, 23.5) -> (-119, 2.5)
  line L29 (-121, 2.5) -> (-133, 2.5) projected
  line L30 (-121, 27) -> (-121, 2.5) projected
  line L31 (-119, -2.5) -> (-118, -2.5)
  line L32 (-118, -2.5) -> (-118, -23.5)
  line L33 (-118, -23.5) -> (-119, -23.5)
  line L34 (-119, -23.5) -> (-119, -2.5)
  line L35 (-133, -2.5) -> (-121, -2.5) projected
  line L36 (-121, -2.5) -> (-121, -27) projected
  point P0 (0, 0)
  point P1 (-53.5, -26.75)
  point P2 (-53.5, -48.75)
  point P3 (-45, -50)
  point P4 (-22.5, -26.75)
  point P5 (-25, -37.75)
  point P6 (-23, -37.75)
  point P7 (-53.5, 47.75)
  point P8 (-22.5, 47.75)
  point P9 (-118.5, 2.5)
  point P10 (-121, 14.75)
  point P11 (-118.5, -2.5)
  dimension "d391" = 1
  dimension "d392" = 22
  dimension "d393" = 1.25
  dimension "d394" = 1.25
  dimension "d395" = 1
  dimension "d396" = 22
  dimension "d397" = 1.25
  dimension "d398" = 2
  dimension "d399" = 2
  dimension "d400" = 1
  dimension "d401" = 20
  dimension "d402" = 1
  dimension "d403" = 20
  dimension "d404" = 2.25
  dimension "d405" = 2.25
  dimension "d406" = 2
  dimension "d407" = 2
  dimension "d408" = 1
  dimension "d409" = 21
  dimension "d410" = 0
  dimension "d411" = 2
  dimension "d412" = 1
  dimension "d413" = 21
  dimension "d414" = 0
  dimension "d415" = 2
  constraints: 48 end point, 12 parallel, 11 midpoint, 6 horizontal, 6 perpendicular
  measures "d391" distance of L2.end L1.end
  measures "d392" distance of L1.end L0.end
  measures "d393" distance from line of L4 point (-53.5, -26.75)
  measures "d394" vertical distance of point (-53.5, -48.75) point (-45, -50)
  measures "d395" distance of L7.end L8.end
  measures "d396" distance of L6.end L7.end
  measures "d397" distance from line of L10 point (-22.5, -26.75)
  measures "d398" distance between parallel lines of L11 L3
  measures "d399" distance of point (-25, -37.75) point (-23, -37.75)
  measures "d400" distance of L15.end L14.end
  measures "d401" distance of L14.end L13.end
  measures "d402" distance of L18.end L19.end
  measures "d403" distance of L17.end L18.end
  measures "d404" distance from line of L21 point (-53.5, 47.75)
  measures "d405" distance from line of L22 point (-22.5, 47.75)
  measures "d406" distance between parallel lines of L23 L20
  measures "d407" distance between parallel lines of L24 L16
  measures "d408" distance of L27.end L26.end
  measures "d409" distance of L26.end L25.end
  measures "d410" distance from line of L29 point (-118.5, 2.5)
  measures "d411" distance from line of point (-121, 14.75) L28
  measures "d412" distance of L32.end L33.end
  measures "d413" distance of L31.end L32.end
  measures "d414" distance from line of L35 point (-118.5, -2.5)
  measures "d415" distance between parallel lines of L36 L34
extrude "Wyciągnięcie proste36" cut sketch "Szkic38" against normal blind 2
